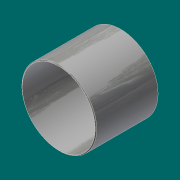
# Autodesk Inventor part: A1-19027-200-xx 36in pipe
Saved by Autodesk Inventor 2017.3 (Build 213256000, 256)
## iProperties
Created: 2019-06-26
Part Number: A1-19027-200-xx 36in pipe
Material: Steel, Mild
Document SubType Name: Modeling
Designer: Graeme_Van_Dongen
Density: 7.85 g/cm^3
Appearance: Steel
Author: Graeme_Van_Dongen
Autodesk Inventor part; units mm, degrees
ref_plane "YZ Plane" through (0, 0, 0) normal (1, 0, 0) x (0, 1, 0)
ref_plane "XZ Plane" through (0, 0, 0) normal (0, 1, 0) x (-1, 0, 0)
ref_plane "XY Plane" through (0, 0, 0) normal (0, 0, 1) x (1, 0, 0)
sketch "Sketch1" plane through (0, 0, 0) normal (0, 0, 1) x (1, 0, 0)
  circle A0 centre (0, 0) radius 457.2
  circle A1 centre (0, 0) radius 444.5
  dimension "d0" = 914.4
  dimension "d1" = 889
  constraints: 2 centre point, 2 coincident
  measures "d0" diameter of A0
  measures "d1" diameter of A1
extrude "Extrusion1" add sketch "Sketch1" along normal blind 766.6
chamfer "Chamfer1" distance 11.1125 angle 37.5 1 edges at (-457.2, 0, 0) measured on face at (-456.7, 0, 0)
chamfer "Chamfer2" distance 11.1125 angle 37.5 1 edges at (-457.2, 0, 766.6) measured on face at (-456.7, 0, 766.6)
equation "\"d7\" = d4"
equation "\"d9\" = d6"
equation "\"d4\" = 11.1125"
equation "\"d6\" = 37.5deg"
body "Solid1"
